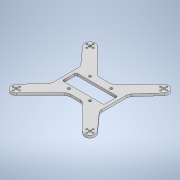
# Autodesk Inventor part: Crazyflie Bolt Mount
Saved by Autodesk Inventor 2021 (Build 250183000, 183)
## iProperties
Created: 2021-06-23
Part Number: Crazyflie Bolt Mount
Material: Generic
Document SubType Name: Modeling
Designer: Gilbert
Density: 1 g/cm^3
Appearance: Default
Author: Gilbert
Autodesk Inventor part; units mm, degrees
ref_plane "YZ Plane" through (0, 0, 0) normal (1, 0, 0) x (0, 1, 0)
ref_plane "XZ Plane" through (0, 0, 0) normal (0, 1, 0) x (-1, 0, 0)
ref_plane "XY Plane" through (0, 0, 0) normal (0, 0, 1) x (1, 0, 0)
sketch "Sketch1" plane through (0, 0, 0) normal (0, 1, 0) x (-1, 0, 0)
  line L0 (15.25, -15.25) -> (-15.25, -15.25)
  line L1 (-15.25, 15.25) -> (15.25, 15.25)
  line L2 (15.25, -15.25) -> (-15.25, 15.25) construction
  line L3 (-15.25, -15.25) -> (15.25, 15.25) construction
  circle A0 centre (15.25, -15.25) radius 1.75
  circle A1 centre (-15.25, -15.25) radius 1.75
  circle A2 centre (15.25, 15.25) radius 1.75
  circle A3 centre (-15.25, 15.25) radius 1.75
  line L4 (21, -15.25) -> (-21, -15.25)
  line L5 (-21, -15.25) -> (-21, 15.25)
  line L6 (-21, 15.25) -> (21, 15.25)
  line L7 (21, 15.25) -> (21, -15.25)
  line L8 (21, -15.25) -> (-21, 15.25) construction
  line L9 (-21, -15.25) -> (21, 15.25) construction
  circle A4 centre (15.25, 15.25) radius 2.5
  circle A5 centre (-15.25, 15.25) radius 2.5
  circle A6 centre (-15.25, -15.25) radius 2.5
  circle A7 centre (15.25, -15.25) radius 2.5
  line L10 (22.5, -17.75) -> (-22.5, -17.75)
  line L11 (-22.5, -17.75) -> (-22.5, 17.75)
  line L12 (-22.5, 17.75) -> (22.5, 17.75)
  line L13 (22.5, 17.75) -> (22.5, -17.75)
  line L14 (22.5, -17.75) -> (-22.5, 17.75) construction
  line L15 (-22.5, -17.75) -> (22.5, 17.75) construction
  point P0 (0, 0)
  point P1 (12.75, 15.25)
  point P2 (17.75, 15.25)
  point P3 (17.75, -15.25)
  point P4 (12.75, -15.25)
  point P5 (-12.75, -15.25)
  point P6 (-17.75, -15.25)
  point P7 (-17.75, 15.25)
  point P8 (-12.75, 15.25)
  dimension "d0" = 30.5
  dimension "d1" = 30.5
  dimension "d2" = 3.5
  dimension "d3" = 3.5
  dimension "d4" = 3.5
  dimension "d5" = 3.5
  dimension "d6" = 42
  dimension "d7" = 5
  dimension "d8" = 5
  dimension "d9" = 5
  dimension "d10" = 5
  dimension "d11" = 45
  constraints: 32 end point, 8 centre point, 7 coincident, 6 midpoint, 5 parallel, 2 horizontal, 2 perpendicular
  measures "d0" distance of L0.start L0.end
  measures "d1" distance of L0.end L1.start
  measures "d2" diameter of A0
  measures "d3" diameter of A1
  measures "d4" diameter of A2
  measures "d5" diameter of A3
  measures "d6" distance of L4.start L4.end
  measures "d7" diameter of A4
  measures "d8" diameter of A5
  measures "d9" diameter of A6
  measures "d10" diameter of A7
  measures "d11" distance of L10.start L10.end
sketch "Sketch2" plane through (0, 0, 0) normal (0, 1, 0) x (-1, 0, 0)
  line L0 (30, -10) -> (-30, -10)
  line L1 (-30, -10) -> (-30, 10)
  line L2 (-30, 10) -> (30, 10)
  line L3 (30, 10) -> (30, -10)
  line L4 (30, -10) -> (-30, 10) construction
  line L5 (-30, -10) -> (30, 10) construction
  line L6 (2.5, -2.5) -> (-2.5, -2.5)
  line L7 (-2.5, -2.5) -> (-2.5, 2.5)
  line L8 (-2.5, 2.5) -> (2.5, 2.5)
  line L9 (2.5, 2.5) -> (2.5, -2.5)
  line L10 (2.5, -2.5) -> (-2.5, 2.5) construction
  line L11 (-2.5, -2.5) -> (2.5, 2.5) construction
  line L12 (0, 0) -> (53.033, 53.033)
  line L13 (0, 0) -> (53.033, -53.033)
  line L14 (0, 0) -> (-53.033, -53.033)
  line L15 (0, 0) -> (-53.033, 53.033)
  circle A0 centre (-53.033, -53.033) radius 32.5
  circle A1 centre (53.033, -53.033) radius 32.5
  circle A2 centre (53.033, 53.033) radius 32.5
  circle A3 centre (-53.033, 53.033) radius 32.5
  circle A4 centre (-53.033, 53.033) radius 7.5
  circle A5 centre (53.033, 53.033) radius 7.5
  circle A6 centre (-53.033, -53.033) radius 7.5
  circle A7 centre (53.033, -53.033) radius 7.5
  line L16 (34.5, 21) -> (-34.5, 21)
  line L17 (-34.5, 21) -> (-34.5, -21)
  line L18 (-34.5, -21) -> (34.5, -21)
  line L19 (34.5, -21) -> (34.5, 21)
  line L20 (34.5, 21) -> (-34.5, -21) construction
  line L21 (-34.5, 21) -> (34.5, -21) construction
  line L22 (34.5, -21) -> (58.6289, -48.0394)
  line L23 (58.6289, -48.0394) -> (47.4371, -58.0266)
  line L24 (47.4371, -58.0266) -> (10.4105, -21)
  line L25 (-34.5, -21) -> (-58.6289, -48.0394)
  line L26 (-47.4371, -58.0266) -> (-10.4105, -21)
  line L27 (-34.5, 21) -> (-58.6289, 48.0394)
  line L28 (-47.4371, 58.0266) -> (-10.4105, 21)
  line L29 (47.4371, 58.0266) -> (10.4105, 21)
  line L30 (34.5, 21) -> (58.6289, 48.0394)
  line L31 (15.25, 15.25) -> (-15.25, 15.25)
  line L32 (-15.25, 15.25) -> (-15.25, -15.25)
  line L33 (-15.25, -15.25) -> (15.25, -15.25)
  line L34 (15.25, -15.25) -> (15.25, 15.25)
  line L35 (15.25, 15.25) -> (-15.25, -15.25) construction
  line L36 (-15.25, 15.25) -> (15.25, -15.25) construction
  circle A8 centre (15.25, -15.25) radius 1.75
  circle A9 centre (-15.25, -15.25) radius 1.75
  circle A10 centre (15.25, 15.25) radius 1.75
  circle A11 centre (-15.25, 15.25) radius 1.75
  circle A12 centre (53.033, 53.033) radius 4.5
  circle A13 centre (-53.033, 53.033) radius 4.5
  circle A14 centre (-53.033, -53.033) radius 4.5
  circle A15 centre (53.033, -53.033) radius 4.5
  line L37 (57.533, 53.033) -> (48.533, 53.033)
  line L38 (53.033, 57.533) -> (53.033, 48.533)
  circle A16 centre (57.533, 53.033) radius 1.25
  circle A17 centre (53.033, 48.533) radius 1.25
  circle A18 centre (48.533, 53.033) radius 1.25
  circle A19 centre (53.033, 57.533) radius 1.25
  circle A20 centre (-53.033, 57.533) radius 1.25
  circle A21 centre (-53.033, 48.533) radius 1.25
  circle A22 centre (-57.533, 53.033) radius 1.25
  circle A23 centre (-48.533, 53.033) radius 1.25
  circle A24 centre (-57.533, -53.033) radius 1.25
  circle A25 centre (-48.533, -53.033) radius 1.25
  circle A26 centre (-53.033, -57.533) radius 1.25
  circle A27 centre (-53.033, -48.533) radius 1.25
  circle A28 centre (48.533, -53.033) radius 1.25
  circle A29 centre (57.533, -53.033) radius 1.25
  circle A30 centre (53.033, -57.533) radius 1.25
  circle A31 centre (53.033, -48.533) radius 1.25
  circle A32 centre (53.033, 53.033) radius 2
  circle A33 centre (-53.033, 53.033) radius 2
  circle A34 centre (-53.033, -53.033) radius 2
  circle A35 centre (53.033, -53.033) radius 2
  dimension "d14" = 60
  dimension "d15" = 20
  dimension "d16" = 5
  dimension "d17" = 5
  dimension "d20" = 75
  dimension "d21" = 75
  dimension "d22" = 75
  dimension "d23" = 65
  dimension "d24" = 65
  dimension "d25" = 65
  dimension "d26" = 65
  dimension "d27" = 75
  dimension "d28" = 15
  dimension "d29" = 15
  dimension "d31" = 15
  dimension "d32" = 15
  dimension "d33" = 69
  dimension "d34" = 42
  dimension "d35" = 30.5
  dimension "d36" = 30.5
  dimension "d37" = 3.5
  dimension "d38" = 3.5
  dimension "d39" = 3.5
  dimension "d40" = 3.5
  dimension "d41" = 9
  dimension "d42" = 9
  dimension "d43" = 9
  dimension "d44" = 9
  dimension "d45" = 2.5
  dimension "d46" = 2.5
  dimension "d47" = 2.5
  dimension "d48" = 2.5
  dimension "d49" = 2.5
  dimension "d50" = 2.5
  dimension "d51" = 2.5
  dimension "d52" = 2.5
  dimension "d53" = 2.5
  dimension "d54" = 2.5
  dimension "d55" = 2.5
  dimension "d56" = 2.5
  dimension "d57" = 2.5
  dimension "d58" = 2.5
  dimension "d59" = 2.5
  dimension "d60" = 2.5
  dimension "d61" = 4
  dimension "d62" = 4
  dimension "d63" = 4
  dimension "d64" = 4
  constraints: 78 end point, 36 centre point, 25 point on circle, 22 coincident, 9 midpoint, 9 perpendicular, 9 point on line, 8 parallel, 4 horizontal, 4 tangent
  measures "d14" distance of L0.start L0.end
  measures "d15" distance of L0.end L1.end
  measures "d16" distance of L6.start L6.end
  measures "d17" distance of L6.end L7.end
  measures "d20" distance of L12.start L12.end
  measures "d21" distance of L12.start L13.end
  measures "d22" distance of L12.start L14.end
  measures "d23" diameter of A0
  measures "d24" diameter of A1
  measures "d25" diameter of A2
  measures "d26" diameter of A3
  measures "d27" distance of L12.start L15.end
  measures "d28" diameter of A4
  measures "d29" diameter of A5
  measures "d31" diameter of A6
  measures "d32" diameter of A7
  measures "d33" distance of L16.start L16.end
  measures "d34" distance of L17.end L16.end
  measures "d35" distance of L31.start L31.end
  measures "d36" distance of L32.end L31.end
  measures "d37" diameter of A8
  measures "d38" diameter of A9
  measures "d39" diameter of A10
  measures "d40" diameter of A11
  measures "d41" diameter of A12
  measures "d42" diameter of A13
  measures "d43" diameter of A14
  measures "d44" diameter of A15
  measures "d45" diameter of A16
  measures "d46" diameter of A17
  measures "d47" diameter of A18
  measures "d48" diameter of A19
  measures "d49" diameter of A20
  measures "d50" diameter of A21
  measures "d51" diameter of A22
  measures "d52" diameter of A23
  measures "d53" diameter of A24
  measures "d54" diameter of A25
  measures "d55" diameter of A26
  measures "d56" diameter of A27
  measures "d57" diameter of A28
  measures "d58" diameter of A29
  measures "d59" diameter of A30
  measures "d60" diameter of A31
  measures "d61" diameter of A32
  measures "d62" diameter of A33
  measures "d63" diameter of A34
  measures "d64" diameter of A35
extrude "Extrusion2" add sketch "Sketch2" along normal blind 3.5 contours L3 L2 L34 A10 L12 L16 L19 L18 L13 A8 L0 | L34 A8 L13 L0 | L13 A8 L33 A9 L14 L0 | L2 L12 A10 L34 | L14 A9 L32 L0 | L2 L15 A11 L31 A10 L12 | L32 A9 L14 L18 L17 L16 L15 A11 L2 L1 L0 | A8 L13 L18 L14 A9 L33 | L2 L32 A11 L15 | L18 L22 A1 L13 | L13 A1 L24 L18 | L31 A11 L15 L16 L12 A10 | A1 L22 A7 L13 | L13 A7 L24 A1 | L16 L29 A2 L12 | L12 A2 L30 L16 | L18 L26 A0 L14 | L14 A0 L25 L18 | A7 L23 A15 A31 L13 | L13 A15 A28 L23 A7 | A2 L29 A5 L12 | L12 A5 L30 A2 | L16 L27 A3 L15 | L15 A3 L28 L16 | A0 L26 A6 L14 | L14 A6 L25 A0 | A15 A31 L23 A35 L13 | L13 A35 L23 A15 A28 | A7 L23 A15 A30 A29 | A12 A18 L37 A32 L12 | L12 A32 L38 A17 A12 | A5 | A3 L27 A4 L15 | L15 A4 L28 A3 | A14 A25 A26 A24 A27 | A6 | A15 A29 A30 L23 A35 | A13 A21 A22 A20 A23 | A4 | L37 A18 A12 A19 L38 A32 | A32 L37 A16 A12 A17 L38 | A32 L38 A19 A12 A16 L37
fillet "Fillet1" radius 8 8 edges at (-10.4105, 1.75, 21) (-34.5, 1.75, 21) (-34.5, 1.75, -21) (34.5, 1.75, -21) (10.4105, 1.75, -21) (10.4105, 1.75, 21) (34.5, 1.75, 21) (-10.4105, 1.75, -21)
fillet "Fillet2" radius 2 4 edges at (-30, 1.75, -10) (30, 1.75, -10) (30, 1.75, 10) (-30, 1.75, 10)
body "Solid2"
